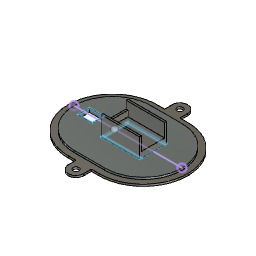
Bell (Autodesk Fusion 360 design; units mm, degrees)
Autodesk Fusion 360 part; units mm, degrees
sketch "Sketch1" plane through (0, 0, 0) normal (0, 0, 1) x (1, 0, 0)
  line L0 (20, 0) -> (36, 0)
  line L1 (56, 20) -> (56, 20)
  line L2 (36, 40) -> (20, 40)
  line L3 (0, 20) -> (0, 20)
  arc A0 (20, 40) -> (0, 20) centre (20, 20) ccw
  arc A1 (56, 20) -> (36, 40) centre (36, 20) ccw
  arc A2 (0, 20) -> (20, 0) centre (20, 20) ccw
  arc A3 (36, 0) -> (56, 20) centre (36, 20) ccw
  point P0 (55, 0)
  point P1 (0, 40)
  dimension "d1" = 55
  dimension "d2" = 40
  dimension "d3" = 20
  dimension "d4" = 20
  dimension "d5" = 20
  dimension "d6" = 20
  constraint horizontal L0
  constraint horizontal L2
  constraint coincident P1 L2
  constraint tangent L2 A0
  constraint tangent L2 A1
  constraint coincident origin L0
  constraint coincident origin L3
  constraint tangent L0 A2
  constraint coincident P0 L0
  constraint coincident P0 L1
  constraint tangent L0 A3
  constraint tangent A0 A2
  constraint tangent A1 A3
  measures "d1" distance of origin P0
  measures "d2" distance of origin P1
  measures "d3" radius of A0
  measures "d4" radius of A1
  measures "d5" radius of A2
  measures "d6" radius of A3
extrude "Extrude1" add sketch "Sketch1" along normal blind 1
sketch "Sketch2" plane through (0, 0, 0) normal (0, 0, -1) x (1, 0, 0)
  arc A0 (36, -40) -> (36, 0) centre (36, -20) ccw
  line L0 (36, 0) -> (20, 0)
  arc A1 (20, 0) -> (20, -40) centre (20, -20) ccw
  line L1 (20, -40) -> (36, -40)
  arc A2 (36, -43) -> (36, 3) centre (36, -20) ccw
  line L2 (36, 3) -> (20, 3)
  arc A3 (20, 3) -> (20, -43) centre (20, -20) ccw
  line L3 (20, -43) -> (36, -43)
  line L4 (28, 0) -> (28, 8) construction
  line L5 (28, 0) -> (24, 0) construction
  line L6 (24, 0) -> (32, 0)
  line L7 (32, 0) -> (32, 7)
  line L8 (28, 11) -> (28, 11)
  line L9 (24, 7) -> (24, 0)
  arc A4 (28, 11) -> (24, 7) centre (28, 7) ccw
  arc A5 (32, 7) -> (28, 11) centre (28, 7) ccw
  line L10 (0, -20) -> (56, -20)
  line L11 (28, -40) -> (28, -48) construction
  line L12 (28, -40) -> (32, -40)
  line L13 (32, -40) -> (24, -40)
  line L14 (24, -40) -> (24, -47)
  line L15 (28, -51) -> (28, -51)
  line L16 (32, -47) -> (32, -40)
  arc A6 (24, -47) -> (28, -51) centre (28, -47) ccw
  arc A7 (28, -51) -> (32, -47) centre (28, -47) ccw
  circle A8 centre (28, 7) radius 1.5
  circle A9 centre (28, -47) radius 1.5
  point P0 (24, 11)
  point P1 (32, -51)
  dimension "d9" = 3
  dimension "d12" = 8
  dimension "d13" = 4
  dimension "d14" = 8
  dimension "d15" = 11
  dimension "d16" = 4
  dimension "d17" = 4
  dimension "d18" = 8
  dimension "d19" = 4
  dimension "d20" = 8
  dimension "d21" = 11
  dimension "d22" = 4
  dimension "d23" = 4
  dimension "d26" = 3
  dimension "d27" = 3
  constraint vertical L4
  constraint midpoint L0 L4.start
  constraint horizontal L5
  constraint horizontal L6
  constraint vertical L7
  constraint vertical L9
  constraint coincident P0 L9
  constraint tangent L9 A4
  constraint tangent L7 A5
  constraint midpoint A1 L10.start
  constraint midpoint A0 L10.end
  constraint vertical L11
  constraint midpoint L1 L11.start
  constraint coincident L1 L12.end
  constraint horizontal L13
  constraint vertical L14
  constraint vertical L16
  constraint tangent L14 A6
  constraint coincident P1 L15
  constraint coincident P1 L16
  constraint tangent L16 A7
  constraint concentric A5 A8
  constraint concentric A6 A9
  measures "d12" distance of L4.start L4.end
  measures "d13" distance of L4.start L5.end
  measures "d14" distance of L5.end L6.end
  measures "d15" distance of L5.end P0
  measures "d16" radius of A4
  measures "d17" radius of A5
  measures "d18" distance of L11.start L11.end
  measures "d19" distance of L11.start L12.end
  measures "d20" distance of L12.end L13.end
  measures "d21" distance of L12.end P1
  measures "d22" radius of A6
  measures "d23" radius of A7
  measures "d26" diameter of A8
  measures "d27" diameter of A9
extrude "Extrude2" add sketch "Sketch2" along normal blind 1 contours A0 A1 L1 L10 L12 L13 | A0 L0 L1 A2 L2 L3 L7 L16 | A0 L0 A1 L6 L10 | L1 L3 L12 L13 L14 L16 | L0 A1 L1 L2 A3 L3 L9 L14 | L0 L2 L6 L7 L9
extrude "Extrude3" add sketch "Sketch2" along normal up to surface (1 mm away) contours L3 L14 L16 A6 A7 | L2 L7 L9 A4 A5 | A8 | A9
extrude "Extrude4" cut sketch "Sketch2" along normal up to surface (1 mm away) contours A8 | A9
sketch "Sketch3" plane through (0, 0, 1) normal (0, 0, 1) x (-1, 0, 0)
  arc A0 (-36, 0) -> (-36, -40) centre (-36, -20) ccw
  line L0 (-36, -40) -> (-20, -40)
  arc A1 (-20, -40) -> (-20, 0) centre (-20, -20) ccw
  line L1 (-20, 0) -> (-36, 0)
  line L2 (0, -20) -> (-56, -20)
  line L3 (-21, -20) -> (-21, -26) construction
  line L4 (-21, -26) -> (-22, -26)
  line L5 (-22, -26) -> (-22, -14)
  line L6 (-22, -14) -> (-21, -14)
  line L7 (-21, -14) -> (-21, -26)
  line L8 (-21, -27) -> (-41, -27)
  line L9 (-41, -27) -> (-41, -26)
  line L10 (-41, -26) -> (-21, -26)
  line L11 (-21, -26) -> (-21, -27)
  line L12 (-21, -14) -> (-41, -14)
  line L13 (-41, -14) -> (-41, -13)
  line L14 (-41, -13) -> (-21, -13)
  line L15 (-21, -13) -> (-21, -14)
  line L16 (-5, -23) -> (-12.5, -23)
  line L17 (-12.5, -23) -> (-12.5, -17)
  line L18 (-12.5, -17) -> (-5, -17)
  line L19 (-5, -17) -> (-5, -23)
  line L20 (-22, -26) -> (-41, -26)
  line L21 (-41, -26) -> (-41, -14)
  line L22 (-41, -14) -> (-22, -14)
  line L23 (-22, -14) -> (-22, -26)
  dimension "d34" = 6
  dimension "d35" = 1
  dimension "d36" = 12
  dimension "d37" = 20
  dimension "d38" = 20
  dimension "d44" = 7.5
  dimension "d45" = 6
  constraint vertical L3
  constraint horizontal L4
  constraint vertical L5
  constraint horizontal L6
  constraint vertical L7
  constraint horizontal L8
  constraint vertical L9
  constraint horizontal L10
  constraint vertical L11
  constraint horizontal L12
  constraint vertical L13
  constraint horizontal L14
  constraint vertical L15
  constraint horizontal L16
  constraint vertical L17
  constraint horizontal L18
  constraint vertical L19
  constraint horizontal L20
  constraint vertical L21
  constraint horizontal L22
  constraint vertical L23
  measures "d34" distance of L3.start L3.end
  measures "d35" distance of L3.end L4.end
  measures "d36" distance of L3.end L6.end
  measures "d37" distance of L8.start L8.end
  measures "d38" distance of L6.end L12.end
  measures "d44" distance of L16.start L16.end
  measures "d45" distance of L16.start L18.end
extrude "Extrude5" add sketch "Sketch3" along normal blind 6 contours L2 L5 L6 L7 L12 L23 | L2 L4 L5 L7 L10 L23
extrude "Extrude6" add sketch "Sketch3" along normal blind 10 contours L4 L8 L9 L10 L11 L20 | L6 L12 L13 L14 L15 L22
extrude "Extrude7" cut sketch "Sketch3" against normal up to surface (2 mm away) contours L2 L16 L17 L19 | L2 L17 L18 L19
extrude "Extrude8" add sketch "Sketch3" along normal blind 3 contours L2 L5 L12 L21 L22 L23 | L2 L5 L10 L20 L21 L23
